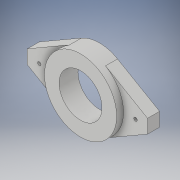
# Autodesk Inventor part: PneumaticHolder
Saved by Autodesk Inventor 2019 (Build 230136000, 136)
## iProperties
Created: 2021-10-31
Part Number: PneumaticHolder
Material: Generic
Document SubType Name: Modeling
Designer: Mohamed Teleb
Density: 1 g/cm^3
Appearance: Default
Author: Mohamed Teleb
Autodesk Inventor part; units mm, degrees
ref_plane "YZ Plane" through (0, 0, 0) normal (1, 0, 0) x (0, 1, 0)
ref_plane "XZ Plane" through (0, 0, 0) normal (0, 1, 0) x (-1, 0, 0)
ref_plane "XY Plane" through (0, 0, 0) normal (0, 0, 1) x (1, 0, 0)
sketch "Sketch1" plane through (0, 0, 0) normal (0, 0, 1) x (1, 0, 0)
  circle A0 centre (0, 0) radius 12.5
  circle A1 centre (0, 0) radius 21
  line L0 (0, 0) -> (-28, 0)
  line L1 (0, 0) -> (28, 0)
  circle A2 centre (-28, 0) radius 1
  circle A3 centre (28, 0) radius 1
  line L2 (0, 0) -> (-35, 0)
  line L3 (0, 0) -> (35, 0)
  line L4 (-35, -4) -> (-35, 4)
  line L5 (35, 4) -> (35, -4)
  line L6 (-35, 4) -> (-10.5231, 18.1732)
  line L7 (-35, -4) -> (-10.5231, -18.1732)
  line L8 (35, 4) -> (10.5231, 18.1732)
  line L9 (35, -4) -> (10.5231, -18.1732)
  dimension "d0" = 25
  dimension "d1" = 42
  dimension "d2" = 28
  dimension "d3" = 28
  dimension "d4" = 2
  dimension "d5" = 2
  dimension "d6" = 35
  dimension "d7" = 35
  dimension "d8" = 8
  dimension "d9" = 4
  dimension "d10" = 8
  dimension "d11" = 4
  constraints: 20 end point, 4 centre point, 4 coincident, 4 point on circle, 3 tangent, 2 horizontal, 2 point on line, 2 vertical, 1 parallel
  measures "d0" diameter of A0
  measures "d1" diameter of A1
  measures "d2" distance of L0.start L0.end
  measures "d3" distance of L0.start L1.end
  measures "d4" diameter of A2
  measures "d5" diameter of A3
  measures "d6" distance of L0.start L2.end
  measures "d7" distance of L0.start L3.end
  measures "d8" distance of L4.start L4.end
  measures "d9" vertical distance of L4.end L0.end
  measures "d10" distance of L5.start L5.end
  measures "d11" vertical distance of L5.start A3.centre
extrude "Extrusion1" add sketch "Sketch1" along normal blind 7 contours L1 A3 L3 L5 L9 A1 | A1 L8 L5 L3 A3 L1 | L0 A2 L2 L4 L6 A1 | A1 L7 L4 L2 A2 L0
sketch "Sketch2" plane through (0, 0, 0) normal (0, 0, -1) x (-1, 0, 0)
  circle A0 centre (0, 0) radius 21
  circle A1 centre (0, 0) radius 12.5
  dimension "d14" = 25
  constraints: 2 centre point, 2 coincident
  measures "d14" diameter of A1
extrude "Extrusion2" add sketch "Sketch2" against normal blind 11
equation "\"d9\" = 0.5 * d8"
equation "\"d11\" = 0.5 * d10"
body "Solid1"
